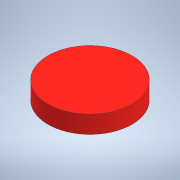
# Autodesk Inventor part: red_lid
Saved by Autodesk Inventor 2021 (Build 250183000, 183)
## iProperties
Created: 2026-10-08
Part Number: red_lid
Material: Generic
Document SubType Name: Modeling
Designer: alolo
Density: 1 g/cm^3
Appearance: Default
Author: alolo
Autodesk Inventor part; units mm, degrees
ref_plane "YZ Plane" through (0, 0, 0) normal (1, 0, 0) x (0, 1, 0)
ref_plane "XZ Plane" through (0, 0, 0) normal (0, 1, 0) x (-1, 0, 0)
ref_plane "XY Plane" through (0, 0, 0) normal (0, 0, 1) x (1, 0, 0)
sketch "Sketch1" plane through (0, 0, 0) normal (0, 0, 1) x (1, 0, 0)
  line L0 (31, 0) -> (31, 13)
  line L1 (31, 13) -> (0, 13)
  line L2 (0, 11.5) -> (29.5, 11.5)
  line L3 (29.5, 11.5) -> (29.5, 0)
  line L4 (0, 11.5) -> (0, 13)
  line L5 (29.5, 0) -> (31, 0)
  line L6 (0, 0) -> (0, 13) construction
  dimension "d8" = 13
  dimension "d9" = 31
  dimension "d10" = 1.5
  constraints: 14 end point, 3 perpendicular, 3 vertical, 1 horizontal alignment, 1 vertical alignment, 1 other
  measures "d8" distance of L0.start L0.end
  measures "d9" distance of L0.end L1.end
  measures "d10" distance between parallel lines of L1 L2
revolve "Revolution1" add sketch "Sketch1" angle 360 about axis through (0, 0, 0) along (0, 1, 0)
body "Solid1"
